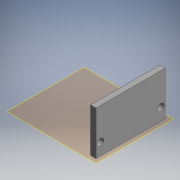
# Autodesk Inventor part: Part15
Saved by Autodesk Inventor 2016 (Build 200138000, 138)
## iProperties
Created: 2018-01-18
Part Number: Part15
Material: Generic
Document SubType Name: Modeling
Designer: student
Density: 1 g/cm^3
Appearance: Default
Author: student
Autodesk Inventor part; units mm, degrees
ref_plane "YZ Plane" through (0, 0, 0) normal (1, 0, 0) x (0, 1, 0)
ref_plane "XZ Plane" through (0, 0, 0) normal (0, 1, 0) x (-1, 0, 0)
ref_plane "XY Plane" through (0, 0, 0) normal (0, 0, 1) x (1, 0, 0)
ref_plane "Work Plane1" through (-108.8053, -23.2276, 20.9918) normal (0, 1, 0) x (-0.9999918, 0, -0.00406)
sketch "Sketch1" plane through (-108.8053, -23.2276, 20.9918) normal (0, 1, 0) x (-0.9999918, 0, -0.00406)
  line L0 (-46.8276, -40.1908) -> (-47.1524, 39.8092) projected
  line L1 (-47.1524, 39.8092) -> (-40.8024, 39.8092)
  line L2 (-46.8276, -40.1908) -> (-40.4776, -40.1908)
  line L3 (-46.8276, -40.1908) -> (-40.4776, -40.1908)
  line L4 (-40.8024, 39.8092) -> (-40.4776, -40.1908)
  point P0 (-108.7192, -21.4334)
  dimension "d0" = 6.35
  dimension "d1" = 6.35
  constraints: 8 end point, 3 horizontal, 1 collinear
  measures "d0" distance of L0.end L1.end
  measures "d1" distance of L0.start L2.end
extrude "Extrusion1" add sketch "Sketch1" along normal blind 50.8
sketch "Sketch2" plane through (-61.8149, -23.2276, 60.9921) normal (1, 0, 0) x (0, 0, -1)
  line L0 (80.0007, 0) -> (0, 0) construction
  line L1 (80.0007, 0) -> (80.0007, 50.8) construction
  line L2 (0, 50.8) -> (80.0007, 50.8) construction
  line L3 (0, 0) -> (0, 50.8) construction
  line L4 (0, 50.8) -> (80.0007, 50.8) construction
  line L5 (40.0003, 50.8) -> (40.0003, 0) construction
  circle A0 centre (5.0003, 13.9978) radius 4
  circle A1 centre (75.0003, 13.9978) radius 4
  line L6 (31.9958, 10.525) -> (47.9958, 10.525) construction
  line L7 (47.9958, 26.375) -> (31.9958, 26.375) construction
  line L8 (47.9958, 26.375) -> (47.9958, 19.525) construction
  line L9 (47.9958, 11.625) -> (47.9958, 10.525) construction
  line L10 (31.9958, 26.375) -> (31.9958, 10.525) construction
  line L11 (47.9958, 26.375) -> (47.9958, 10.525) construction
  line L12 (31.9958, 18.45) -> (47.9958, 18.45) construction
  line L13 (30.3958, 8.94) -> (49.5958, 8.94)
  line L14 (49.5958, 8.94) -> (49.5958, 27.96)
  line L15 (49.5958, 27.96) -> (30.3958, 27.96)
  line L16 (30.3958, 27.96) -> (30.3958, 8.94)
  line L17 (31.9958, 10.525) -> (47.9958, 26.375) construction
  line L18 (47.9958, 10.525) -> (31.9958, 26.375) construction
  point P0 (60.9921, 23.2276)
  point P1 (39.9958, 18.45)
  dimension "d9" = 8
  dimension "d10" = 8
  constraints: 24 end point, 7 midpoint, 2 centre point, 2 parallel, 2 perpendicular, 2 vertical, 1 horizontal, 2 other
  measures "d9" diameter of A0
  measures "d10" diameter of A1
extrude "Extrusion2" cut sketch "Sketch2" against normal blind 50.8
body "Solid1"
